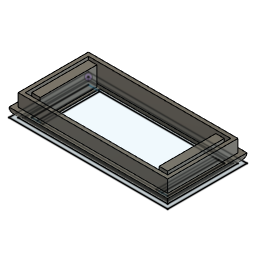
outer_led_panel_frame (Autodesk Fusion 360 design; units mm, degrees)
Autodesk Fusion 360 part; units mm, degrees
sketch "Sketch1" plane through (0, 0, 0) normal (0, 1, 0) x (1, 0, 0)
  line L0 (0, 0) -> (66, 0)
  line L1 (66, 0) -> (66, -31)
  line L2 (66, -31) -> (0, -31)
  line L3 (0, -31) -> (0, 0)
  line L4 (1, -1) -> (65, -1)
  line L5 (65, -1) -> (65, -30)
  line L6 (65, -30) -> (1, -30)
  line L7 (1, -30) -> (1, -1)
  line L8 (63, -28) -> (3, -28)
  line L9 (3, -28) -> (3, -3)
  line L10 (3, -3) -> (63, -3)
  line L11 (63, -3) -> (63, -28)
  line L12 (1.6, -1.6) -> (64.4, -1.6)
  line L13 (64.4, -1.6) -> (64.4, -29.4)
  line L14 (64.4, -29.4) -> (1.6, -29.4)
  line L15 (1.6, -29.4) -> (1.6, -1.6)
  line L16 (68, 2) -> (68, -33)
  line L17 (68, -33) -> (-2, -33)
  line L18 (-2, -33) -> (-2, 2)
  line L19 (-2, 2) -> (68, 2)
  line L20 (3, -28) -> (8, -28)
  line L21 (8, -28) -> (8, -3)
  line L22 (8, -3) -> (3, -3)
  line L23 (3, -3) -> (3, -28)
  line L24 (63, -28) -> (58, -28)
  line L25 (58, -28) -> (58, -3)
  line L26 (58, -3) -> (63, -3)
  line L27 (63, -3) -> (63, -28)
  line L28 (3, -3) -> (5.5, -3)
  line L29 (5.5, -3) -> (5.5, -28)
  line L30 (5.5, -28) -> (3, -28)
  line L31 (3, -28) -> (3, -3)
  line L32 (63, -3) -> (60.5, -3)
  line L33 (60.5, -3) -> (60.5, -28)
  line L34 (60.5, -28) -> (63, -28)
  line L35 (63, -28) -> (63, -3)
  line L36 (5.5, -3) -> (6.75, -3)
  line L37 (6.75, -3) -> (6.75, -28)
  line L38 (6.75, -28) -> (5.5, -28)
  line L39 (5.5, -28) -> (5.5, -3)
  line L40 (60.5, -3) -> (59.25, -3)
  line L41 (59.25, -3) -> (59.25, -28)
  line L42 (59.25, -28) -> (60.5, -28)
  line L43 (60.5, -28) -> (60.5, -3)
  dimension "d1" = 66
  dimension "d2" = 31
  dimension "d3" = 1
  dimension "d4" = 3
  dimension "d5" = 1.6
  dimension "d6" = -2
  dimension "d13" = 5
  dimension "d14" = 5
  dimension "d15" = 25
  dimension "d18" = 2.5
  dimension "d19" = 2.5
  dimension "d24" = 1.25
  dimension "d25" = 1.25
  constraint horizontal L0
  constraint vertical L1
  constraint horizontal L2
  constraint vertical L3
  constraint coincident L0.start L3.end
  constraint horizontal L20
  constraint vertical L21
  constraint horizontal L22
  constraint vertical L23
  constraint horizontal L24
  constraint vertical L25
  constraint horizontal L26
  constraint vertical L27
  constraint horizontal L28
  constraint vertical L29
  constraint horizontal L30
  constraint vertical L31
  constraint horizontal L32
  constraint vertical L33
  constraint horizontal L34
  constraint vertical L35
  constraint horizontal L36
  constraint vertical L37
  constraint horizontal L38
  constraint vertical L39
  constraint horizontal L40
  constraint vertical L41
  constraint horizontal L42
  constraint vertical L43
  measures "d1" distance of L0.start L0.end
  measures "d2" distance of L0.start L2.end
  measures "d13" distance of L8.end L20.end
  measures "d14" distance of L8.start L24.end
  measures "d15" distance of L8.start L10.end
  measures "d18" distance of L9.end L28.end
  measures "d19" distance of L10.end L32.end
  measures "d24" distance of L28.end L36.end
  measures "d25" distance of L32.end L40.end
extrude "Extrude2" add sketch "Sketch1" along normal blind 9.5 contours L0 L1 L2 L3 | L4 L5 L6 L7 | L8 L10 L11 L24 L26 L27 L32 L33 L34 L35 L43 | L8 L10 L24 L26 L33 L40 L41 L42 L43 | L8 L10 L20 L22 L29 L36 L37 L38 L39 | L8 L9 L10 L20 L22 L23 L28 L29 L30 L31 L39 makes body 1 at (22, 6.3333, 0) makes body 2 at (63, 3.1667, 11.3333) makes body 3 at (6.75, 3.1667, 11.3333)
extrude "Extrude1" add sketch "Sketch1" along normal blind 1 contours L8 L10 L24 L26 L33 L40 L41 L42 L43 | L8 L10 L24 L25 L26 L41 | L8 L10 L20 L21 L22 L37 | L8 L10 L20 L22 L29 L36 L37 L38 L39 | L12 L13 L14 L15 bodies 1 2 3
fillet "Fillet2" radius 1 4 edges at (33, 0, 28) (8, 0, 15.5) (33, 0, 3) (58, 0, 15.5) on bodies 1
extrude "Extrude3" add sketch "Sketch1" along normal blind 4 contours L16 L17 L18 L19 bodies 1
fillet "Fillet3" radius 4 4 edges at (-2, 0, 15.5) (33, 0, 33) (33, 0, -2) (68, 0, 15.5) on bodies 1
